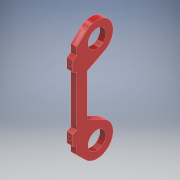
# Autodesk Inventor part: PlateConnector
Saved by Autodesk Inventor 2022 (Build 260153000, 153)
## iProperties
Created: 2021-04-25
Part Number: PlateConnector
Material: Generic
Document SubType Name: Modeling
Designer: Mick Veldhuis
Density: 1 g/cm^3
Appearance: Red
Author: Mick Veldhuis
Autodesk Inventor part; units mm, degrees
ref_plane "YZ Plane" through (0, 0, 0) normal (1, 0, 0) x (0, 1, 0)
ref_plane "XZ Plane" through (0, 0, 0) normal (0, 1, 0) x (-1, 0, 0)
sketch "Sketch1" plane through (0, 0, 0) normal (1, 0, 0) x (0, 1, 0)
  arc A0 (59.469, -14.4909) -> (110.9653, 22.2844) centre (87.9998, 0.0002) ccw
  line L0 (110.9653, 22.2844) -> (93.7688, 40.0067)
  line L1 (0.3424, 140.3326) -> (0.3424, -179.6674) construction
  arc A1 (-110.2805, 22.2844) -> (-58.7842, -14.4909) centre (-87.315, 0.0002) ccw
  line L2 (-110.2805, 22.2844) -> (-93.0839, 40.0067)
  line L3 (-88, 40.0067) -> (-88.0045, 40)
  line L4 (57.9955, 40) -> (58, 40.0067)
  line L5 (49.9965, 40.0151) -> (-50.0337, 40.0151)
  line L6 (59.469, -14.4909) -> (41.9609, 19.9801)
  line L7 (-58.7842, -14.4909) -> (-41.2761, 19.9801)
  line L8 (41.9609, 19.9801) -> (-41.2761, 19.9801)
  line L9 (78, 40.0067) -> (73.9965, 48.0084)
  line L10 (73.9965, 48.0084) -> (53.9965, 48.0084)
  line L11 (53.9965, 48.0084) -> (49.9965, 40.0151)
  line L12 (-78, 40.0067) -> (-74.0035, 48.0084)
  line L13 (-74.0035, 48.0084) -> (-54.0035, 48.0084)
  line L14 (-54.0035, 48.0084) -> (-50.0337, 40.0151)
  line L15 (93.7688, 40.0067) -> (78, 40.0067)
  line L16 (-78, 40.0067) -> (-93.0839, 40.0067)
  point P0 (0, 0)
  point P1 (83, 40)
  point P2 (63.9965, 48.0084)
  point P3 (-64.0035, 48.0084)
  constraints: 34 end point, 6 horizontal, 4 point on circle, 4 symmetric about line, 2 centre point, 2 midpoint, 2 tangent, 1 vertical, 1 other
extrude "Extrusion2" add sketch "Sketch1" along normal blind 12
hole "Hole4" at (0, -87.315, 0.0002) at (0, 87.9998, 0.0002) direction (1, 0, 0) diameter 36 end through all
ref_plane "Work Plane2" through (0, -64.0035, 48.0084) normal (0, 0, 1) x (1, 0, 0)
sketch "Sketch3" plane through (0, -74.0035, 48.0084) normal (0, 0, 1) x (1, 0, 0)
  point P0 (0, 74.0035)
  point P1 (6, 10)
  point P2 (6, 138)
hole "Hole5" at (6, -64.0035, 48.0084) at (6, 63.9965, 48.0084) direction (0, 0, -1) diameter 6.647 depth 20 tip angle 118 thread size "M8x1.25" class "6H" standard "ISO Metric profile"
body "Solid2"
